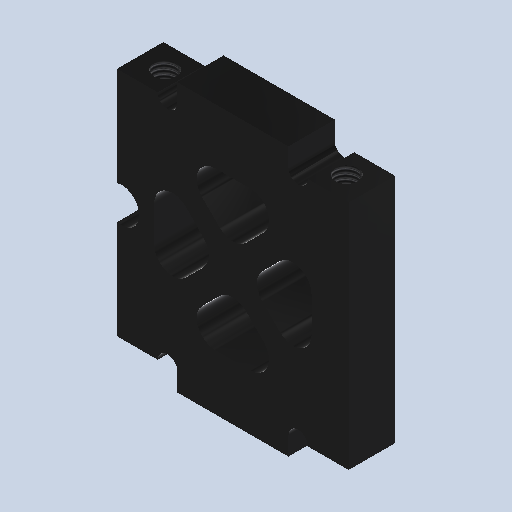
# Autodesk Inventor part: Head_diagonal
Saved by Autodesk Inventor 2022.4 (Build 264492000, 492)
## iProperties
Part Number: Head_diagonal
Material: アセタール樹脂、黒
Document SubType Name: Modeling
Designer: Masato Kubotera
Density: 1.425 g/cm^3
Appearance: 滑らか - 黒
Mass: 3.46837 g
Surface Area: 23.2809 cm^2
Volume: 2.43394 cm^3
Description: POM T5
d0: 25.000 mm
d1: 1.050 mm
d2: 2.000 mm
d3: 6.500 mm
d9: 2.500 mm
d10: 2.500 mm
d11: 2.500 mm
d12: 2.500 mm
d13: 4.000 mm
d14: 2.500 mm
d15: 0.00 deg
d21: 6.000 mm
d25: 8.800 mm
d27: 2.000 ul
d28: 360.00 deg
d30: 2.000 mm
Author: Masato Kubotera
Autodesk Inventor part; units mm, degrees
ref_plane "YZ Plane" through (0, 0, 0) normal (1, 0, 0) x (0, 1, 0)
ref_plane "XZ Plane" through (0, 0, 0) normal (0, 1, 0) x (-1, 0, 0)
ref_plane "XY Plane" through (0, 0, 0) normal (0, 0, 1) x (1, 0, 0)
sketch "スケッチ1" plane through (0, 0, 0) normal (0, 0, 1) x (1, 0, 0)
  line L0 (-12.5, -12.5) -> (12.5, -12.5) construction
  line L1 (12.5, -12.5) -> (12.5, 12.5)
  line L2 (12.5, 12.5) -> (-12.5, 12.5) construction
  line L3 (-12.5, 12.5) -> (-12.5, -12.5)
  line L4 (-12.5, -12.5) -> (12.5, 12.5) construction
  line L5 (12.5, -12.5) -> (-12.5, 12.5) construction
  line L6 (-8.1, 12.5) -> (-12.5, 12.5)
  line L7 (8.1, 12.5) -> (12.5, 12.5)
  line L8 (-12.5, -12.5) -> (-8.1, -12.5)
  line L9 (8.1, -12.5) -> (12.5, -12.5)
  line L10 (-6, 12.5) -> (-6, 14.5)
  line L11 (-6, 14.5) -> (6, 14.5)
  line L12 (6, 14.5) -> (6, 12.5)
  arc A0 (-8.1, 12.5) -> (-6, 12.5) centre (-7.05, 12.5) ccw
  arc A1 (6, 12.5) -> (8.1, 12.5) centre (7.05, 12.5) ccw
  line L13 (0, 12.5) -> (0, 0) construction
  line L14 (0, 0) -> (12.5, 0) construction
  line L15 (-6, -12.5) -> (-6, -14.5)
  line L16 (-6, -14.5) -> (6, -14.5)
  line L17 (6, -14.5) -> (6, -12.5)
  arc A2 (-6, -12.5) -> (-8.1, -12.5) centre (-7.05, -12.5) ccw
  arc A3 (8.1, -12.5) -> (6, -12.5) centre (7.05, -12.5) ccw
  line L18 (-9.05, 12.5) -> (-5.95, 12.5) construction
  line L19 (-6.7322, 8.5) -> (6.7322, 8.5)
  line L20 (6.7322, 8.5) -> (0, 1.7678)
  line L21 (0, 1.7678) -> (-6.7322, 8.5)
  line L22 (-8.5, 6.7322) -> (-8.5, -6.7322)
  line L23 (-8.5, -6.7322) -> (-1.7678, 0)
  line L24 (-1.7678, 0) -> (-8.5, 6.7322)
  line L25 (-6.7322, -8.5) -> (6.7322, -8.5)
  line L26 (6.7322, -8.5) -> (0, -1.7678)
  line L27 (0, -1.7678) -> (-6.7322, -8.5)
  line L28 (8.5, 6.7322) -> (8.5, -6.7322)
  line L29 (8.5, -6.7322) -> (1.7678, 0)
  line L30 (1.7678, 0) -> (8.5, 6.7322)
  line L31 (12.5, 0) -> (12.3, 0)
  arc A4 (-12.5, -1.833) -> (-12.5, 1.833) centre (-12, 0) ccw
  point P0 (-12.5, 0)
  dimension "d0" = 25
  dimension "d1" = 1.05
  dimension "d2" = 2
  dimension "d3" = 6.5
  dimension "d9" = 2.5
  dimension "d10" = 2.5
  dimension "d11" = 2.5
  dimension "d12" = 2.5
  dimension "d13" = 4
  dimension "d31" = 25
  dimension "d44" = 1.9
  dimension "d46" = 0.5
  constraints: 64 end point, 10 point on circle, 8 parallel, 7 horizontal, 5 centre point, 5 midpoint, 5 perpendicular, 4 collinear, 4 horizontal alignment, 4 point on line, 4 symmetric about line, 4 tangent, 4 vertical, 3 equal length, 2 equal radius, 6 other
  measures "d0" distance of L2.end L0.start
  measures "d1" radius of A0
  measures "d2" distance between parallel lines of L2 L11
  measures "d3" distance between parallel lines of L3 L10
  measures "d9" distance between parallel lines of L26 L29
  measures "d10" distance between parallel lines of L24 L21
  measures "d11" distance between parallel lines of L30 L20
  measures "d12" distance between parallel lines of L27 L23
  measures "d13" distance between parallel lines of L19 L2
  measures "d31" distance of L1.end L2.end
  measures "d44" radius of A4
  measures "d46" distance from line of L3 A4.centre
extrude "押し出し1" add sketch "スケッチ1" along normal blind 2.5 contours L9 A3 L17 L16 L15 A2 L8 L3 A4 L6 A0 L10 L11 L12 A1 L7 L1
mirror "ミラー1" about plane through (0, 0, 0) normal (0, 0, -1) of "押し出し1"
sketch "スケッチ2" plane through (-12.5, -12.5, 2.5) normal (0, -1, 0) x (1, 0, 0)
  line L0 (6.5, 0) -> (18.5, 0) construction
  line L1 (12.5, 0) -> (12.5, -5) construction
  line L2 (0, -5) -> (4.4, -5) projected
  line L3 (20.6, -5) -> (25, -5) projected
  line L4 (0, -5) -> (0, 0) projected
  line L5 (25, -5) -> (25, 0) projected
  point P0 (12.5, -2.5)
  point P1 (2.7, -2.5)
  point P2 (22.3, -2.5)
  dimension "d35" = 2.5
  dimension "d37" = 2.5
  dimension "d47" = 2.7
  dimension "d48" = 2.7
  constraints: 2 end point, 1 midpoint, 1 vertical
  measures "d35" distance from line of L2 point (2.7, -2.5)
  measures "d37" distance from line of L3 point (22.3, -2.5)
  measures "d47" distance from line of point (2.7, -2.5) L4
  measures "d48" distance from line of point (22.3, -2.5) L5
hole "穴1" at (-9.8, -12.5, 0) at (9.8, -12.5, 0) direction (0, 1, 0) diameter 2.459 depth 8.8 thread size "M3x0.5" class "6H" standard "ISO Metric profile"
pattern_circular "円形状パターン1" count 2 over 360 about axis through (0, 0, -10) along (0, 0, 1) of "穴1"
fillet "フィレット1" radius 2 12 edges at (8.5, 6.7322, 0) (8.5, -6.7322, 0) (6.7322, -8.5, 0) (0, 1.7678, 0) (-1.7678, 0, 0) (-6.7322, -8.5, 0) (-8.5, -6.7322, 0) (6.7322, 8.5, 0) (-8.5, 6.7322, 0) (-6.7322, 8.5, 0) (0, -1.7678, 0) (1.7678, 0, 0)
equation "\"d10\" = d9"
equation "\"d11\" = d10"
equation "\"d12\" = d11"
